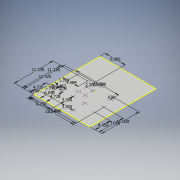
# Autodesk Inventor part: PDU_chassis_bottom
Saved by Autodesk Inventor 2017 (Build 210142000, 142)
## iProperties
Created: 2017-02-14
Part Number: PDU_chassis_bottom
Material: Generic
Document SubType Name: Modeling
Designer: Zara
Density: 1 g/cm^3
Appearance: Default
Author: Zara
Autodesk Inventor part; units mm, degrees
ref_plane "YZ Plane" through (0, 0, 0) normal (1, 0, 0) x (0, 1, 0)
ref_plane "XZ Plane" through (0, 0, 0) normal (0, 1, 0) x (-1, 0, 0)
ref_plane "XY Plane" through (0, 0, 0) normal (0, 0, 1) x (1, 0, 0)
sketch "Sketch1" plane through (0, 0, 0) normal (0, 1, 0) x (-1, 0, 0)
  line L0 (-208.915, 245.999) -> (208.915, 245.999)
  line L1 (208.915, 245.999) -> (208.915, -245.999)
  line L2 (208.915, -245.999) -> (-208.915, -245.999)
  line L3 (-208.915, -245.999) -> (-208.915, 245.999)
  line L4 (-208.915, 245.999) -> (208.915, -245.999) construction
  line L5 (208.915, 245.999) -> (-208.915, -245.999) construction
  point P0 (0, 0)
  dimension "d0" = 491.998
  dimension "d1" = 417.83
  constraints: 12 end point, 2 midpoint, 2 parallel, 1 horizontal, 1 perpendicular
  measures "d0" distance of L2.end L0.start
  measures "d1" distance of L1.end L2.end
extrude "PDU bottom" add sketch "Sketch1" along normal blind 1.651
sketch "Sketch2" plane through (0, 1.651, 0) normal (0, 1, 0) x (1, 0, 0)
  line L0 (-208.915, 245.999) -> (-208.915, -245.999) projected
  line L1 (-208.915, -245.999) -> (208.915, -245.999) projected
  point P0 (0, 0)
  point P1 (-50.165, -201.549)
  point P2 (38.735, -201.549)
  point P3 (-50.165, -112.649)
  point P4 (38.735, -112.649)
  dimension "d4" = 158.75
  dimension "d5" = 44.45
  dimension "d9" = 88.9
  dimension "d12" = 88.9
  constraints: 1 horizontal, 1 vertical, 3 other
  measures "d4" distance from line of L0 point (-50.165, -201.549)
  measures "d5" distance from line of point (-50.165, -201.549) L1
  measures "d9" distance of point (-50.165, -201.549) point (38.735, -201.549)
  measures "d12" distance of point (-50.165, -201.549) point (-50.165, -112.649)
sketch "Sketch3" plane through (0, 1.651, 0) normal (0, 1, 0) x (1, 0, 0)
  line L0 (-208.915, 245.999) -> (-208.915, -245.999) projected
  line L1 (-208.915, -245.999) -> (208.915, -245.999) projected
  point P0 (0, 0)
  point P1 (135.001, -132.7404)
  point P2 (135.001, -67.7418)
  dimension "d22" = 343.916
  dimension "d23" = 113.2586
  dimension "d24" = 178.2572
  dimension "d25" = 343.916
  measures "d22" distance from line of L0 point (135.001, -132.74)
  measures "d23" distance from line of point (135.001, -132.74) L1
  measures "d24" distance from line of point (135.001, -67.742) L1
  measures "d25" distance from line of point (135.001, -67.742) L0
sketch "Sketch4" plane through (0, 1.651, 0) normal (0, 1, 0) x (1, 0, 0)
  line L0 (-208.915, 245.999) -> (-208.915, -245.999) projected
  line L1 (-208.915, -245.999) -> (208.915, -245.999) projected
  line L2 (208.915, -245.999) -> (208.915, 245.999) projected
  line L3 (208.915, 245.999) -> (-208.915, 245.999) projected
  line L4 (-208.915, 245.999) -> (-208.915, -245.999) projected
  point P0 (0, 0)
  point P1 (-58.928, 56.896)
  point P2 (-58.928, -1.524)
  point P3 (-58.928, -59.944)
  point P4 (-11.176, 56.896)
  point P5 (-11.176, -1.524)
  point P6 (-11.176, -59.944)
  dimension "d33" = 149.987
  dimension "d36" = 58.42
  dimension "d39" = 47.752
  dimension "d65" = 302.895
  constraints: 1 horizontal, 1 vertical, 5 other
  measures "d33" distance from line of L0 point (-58.928, 56.896)
  measures "d36" distance of point (-58.928, 56.896) point (-58.928, -1.524)
  measures "d39" distance of point (-58.928, 56.896) point (-11.176, 56.896)
  measures "d65" distance from line of L1 point (-58.928, 56.896)
sketch "Sketch6" plane through (0, 0, 0) normal (0, -1, 0) x (1, 0, 0)
  line L0 (208.915, 245.999) -> (-208.915, 245.999) projected
  line L1 (-208.915, 245.999) -> (-208.915, -245.999) projected
  line L2 (-208.915, -245.999) -> (208.915, -245.999) projected
  line L3 (208.915, -245.999) -> (208.915, 245.999) projected
  point P0 (0, 0)
  point P1 (-11.176, 1.524)
  point P2 (-11.176, 59.944)
  point P3 (-58.928, 59.944)
  point P4 (-58.928, 1.524)
  point P5 (-58.928, -56.896)
  point P6 (-11.176, -56.896)
hole "enable holes" at (-11.176, 0, 1.524) at (-11.176, 0, 59.944) at (-58.928, 0, 59.944) at (-58.928, 0, 1.524) at (-58.928, 0, -56.896) at (-11.176, 0, -56.896) direction (0, 1, 0) diameter 3.4036 end through all countersink diameter 6.2992 countersink angle 90 clearance for "Flat Head Machine Screw" size "M3" standard "Ansi Metric M Profile"
sketch "Sketch7" plane through (0, 0, 0) normal (0, -1, 0) x (1, 0, 0)
  circle A0 centre (-58.928, -56.896) radius 3.1496 projected
  circle A1 centre (-58.928, 59.944) radius 3.1496 projected
  circle A2 centre (-11.176, 1.524) radius 3.1496 projected
  circle A3 centre (-11.176, 59.944) radius 3.1496 projected
  circle A4 centre (-58.928, 1.524) radius 3.1496 projected
  circle A5 centre (-11.176, -56.896) radius 3.1496 projected
  line L0 (208.915, 245.999) -> (-208.915, 245.999) projected
  line L1 (-208.915, 245.999) -> (-208.915, -245.999) projected
  line L2 (-208.915, -245.999) -> (208.915, -245.999) projected
  line L3 (208.915, -245.999) -> (208.915, 245.999) projected
  point P0 (0, 0)
  point P1 (-50.165, 112.649)
  point P2 (38.735, 112.649)
  point P3 (38.735, 201.549)
  point P4 (-50.165, 201.549)
hole "Inteface circuit board holes" at (38.735, 0, 112.649) at (-50.165, 0, 112.649) at (-50.165, 0, 201.549) at (38.735, 0, 201.549) direction (0, 1, 0) diameter 3.4036 end through all countersink diameter 6.2992 countersink angle 90
sketch "Sketch9" plane through (0, 0, 0) normal (0, -1, 0) x (1, 0, 0)
  circle A0 centre (-50.165, 201.549) radius 3.1496 projected
  circle A1 centre (38.735, 112.649) radius 3.1496 projected
  circle A2 centre (-50.165, 112.649) radius 3.1496 projected
  circle A3 centre (38.735, 201.549) radius 3.1496 projected
  circle A4 centre (-58.928, -56.896) radius 3.1496 projected
  circle A5 centre (-58.928, 59.944) radius 3.1496 projected
  circle A6 centre (-11.176, 1.524) radius 3.1496 projected
  circle A7 centre (-11.176, 59.944) radius 3.1496 projected
  circle A8 centre (-58.928, 1.524) radius 3.1496 projected
  circle A9 centre (-11.176, -56.896) radius 3.1496 projected
  line L0 (208.915, 245.999) -> (-208.915, 245.999) projected
  line L1 (-208.915, 245.999) -> (-208.915, -245.999) projected
  line L2 (-208.915, -245.999) -> (208.915, -245.999) projected
  line L3 (208.915, -245.999) -> (208.915, 245.999) projected
  point P0 (0, 0)
  point P1 (135.001, 67.7418)
  point P2 (135.001, 132.7404)
hole "snap psu holes" at (135.001, 0, 67.7418) at (135.001, 0, 132.7404) direction (0, 1, 0) diameter 3.4036 end through all countersink diameter 6.2992 countersink angle 90 clearance for "Countersunk Flat Head Screw ISO 2009/7046" size "M3" standard "ISO"
sketch "Sketch10" plane through (0, 1.651, 0) normal (0, 1, 0) x (1, 0, 0)
  line L0 (110.871, 33.401) -> (110.871, 9.5758) construction
  line L1 (-208.915, 245.999) -> (-208.915, -245.999) construction
  line L2 (-208.915, -245.999) -> (208.915, -245.999) construction
  point P0 (0, 0)
  dimension "d101" = 319.786
  dimension "d102" = 279.4
  dimension "d103" = 23.8252
  constraints: 2 end point, 1 vertical
  measures "d101" distance from line of L1 L0.start
  measures "d102" distance from line of L2 L0.start
  measures "d103" distance of L0.end L0.start
sketch "Sketch11" plane through (0, 0, 0) normal (0, -1, 0) x (1, 0, 0)
  circle A0 centre (135.001, 67.7418) radius 3.1496 projected
  circle A1 centre (135.001, 132.7404) radius 3.1496 projected
  circle A2 centre (-50.165, 201.549) radius 3.1496 projected
  circle A3 centre (38.735, 112.649) radius 3.1496 projected
  circle A4 centre (-50.165, 112.649) radius 3.1496 projected
  circle A5 centre (38.735, 201.549) radius 3.1496 projected
  circle A6 centre (-58.928, -56.896) radius 3.1496 projected
  circle A7 centre (-58.928, 59.944) radius 3.1496 projected
  circle A8 centre (-11.176, 1.524) radius 3.1496 projected
  circle A9 centre (-11.176, 59.944) radius 3.1496 projected
  circle A10 centre (-58.928, 1.524) radius 3.1496 projected
  circle A11 centre (-11.176, -56.896) radius 3.1496 projected
  line L0 (208.915, 245.999) -> (-208.915, 245.999) projected
  line L1 (-208.915, 245.999) -> (-208.915, -245.999) projected
  line L2 (-208.915, -245.999) -> (208.915, -245.999) projected
  line L3 (208.915, -245.999) -> (208.915, 245.999) projected
  point P0 (0, 0)
  point P1 (110.871, -33.401)
  point P2 (110.871, -9.5758)
hole "thermostat holes" at (110.871, 0, -33.401) at (110.871, 0, -9.5758) direction (0, 1, 0) diameter 3.4 end through all countersink diameter 6.3 countersink angle 90 clearance for "Countersunk Flat Head Screw ISO 2009/7046" size "M3" standard "ISO"
sketch "Sketch12" plane through (0, 1.651, 0) normal (0, 1, 0) x (1, 0, 0)
  line L0 (-208.915, -245.999) -> (208.915, -245.999) projected
  line L1 (-208.915, 245.999) -> (-208.915, -245.999) projected
  point P0 (0, 0)
  point P1 (-173.5074, 41.91)
  point P2 (-94.5134, 41.91)
  point P3 (-173.5074, -126.111)
  point P4 (-122.5042, -126.111)
  point P5 (-134.0104, -91.1098)
  dimension "d111" = 287.909
  dimension "d112" = 287.909
  dimension "d113" = 35.4076
  dimension "d114" = 114.4016
  dimension "d115" = 119.888
  dimension "d116" = 86.4108
  dimension "d117" = 35.4076
  dimension "d118" = 119.888
  dimension "d119" = 154.8892
  dimension "d120" = 74.9046
  measures "d111" distance from line of point (-173.507, 41.91) L0
  measures "d112" distance from line of L0 point (-94.513, 41.91)
  measures "d113" distance from line of point (-173.507, 41.91) L1
  measures "d114" distance from line of L1 point (-94.513, 41.91)
  measures "d115" distance from line of L0 point (-173.507, -126.111)
  measures "d116" distance from line of L1 point (-122.504, -126.111)
  measures "d117" distance from line of L1 point (-173.507, -126.111)
  measures "d118" distance from line of L0 point (-122.504, -126.111)
  measures "d119" distance from line of L0 point (-134.01, -91.11)
  measures "d120" distance from line of L1 point (-134.01, -91.11)
sketch "Sketch13" plane through (0, 0, 0) normal (0, -1, 0) x (1, 0, 0)
  circle A0 centre (110.871, -33.401) radius 3.15 projected
  circle A1 centre (110.871, -9.5758) radius 3.15 projected
  circle A2 centre (135.001, 67.7418) radius 3.1496 projected
  circle A3 centre (135.001, 132.7404) radius 3.1496 projected
  circle A4 centre (-50.165, 201.549) radius 3.1496 projected
  circle A5 centre (38.735, 112.649) radius 3.1496 projected
  circle A6 centre (-50.165, 112.649) radius 3.1496 projected
  circle A7 centre (38.735, 201.549) radius 3.1496 projected
  circle A8 centre (-58.928, -56.896) radius 3.1496 projected
  circle A9 centre (-58.928, 59.944) radius 3.1496 projected
  circle A10 centre (-11.176, 1.524) radius 3.1496 projected
  circle A11 centre (-11.176, 59.944) radius 3.1496 projected
  circle A12 centre (-58.928, 1.524) radius 3.1496 projected
  circle A13 centre (-11.176, -56.896) radius 3.1496 projected
  line L0 (208.915, 245.999) -> (-208.915, 245.999) projected
  line L1 (-208.915, 245.999) -> (-208.915, -245.999) projected
  line L2 (-208.915, -245.999) -> (208.915, -245.999) projected
  line L3 (208.915, -245.999) -> (208.915, 245.999) projected
  point P0 (0, 0)
  point P1 (-173.5074, 126.111)
  point P2 (-122.5042, 126.111)
  point P3 (-134.0104, 91.1098)
  point P4 (-173.5074, -41.91)
  point P5 (-94.5134, -41.91)
hole "Hole11" at (-94.5134, 0, -41.91) at (-173.5074, 0, -41.91) at (-134.0104, 0, 91.1098) at (-173.5074, 0, 126.111) at (-122.5042, 0, 126.111) direction (0, 1, 0) diameter 3.4 end through all countersink diameter 6.3 countersink angle 90 clearance for "Countersunk Flat Head Screw ISO 2009/7046" size "M3" standard "ISO"
body "Solid1"
